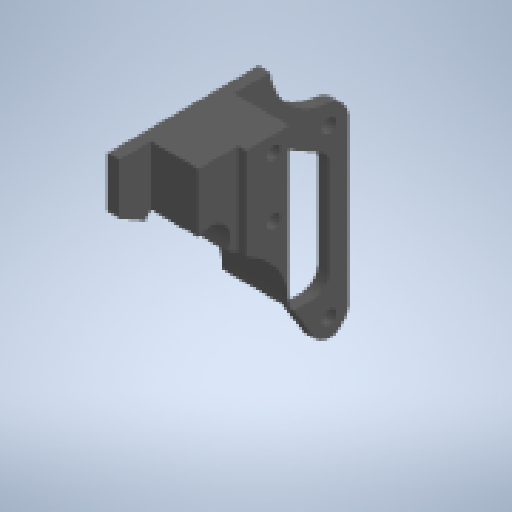
# Autodesk Inventor part: toe_springjoint_bace_upper_left
Saved by Autodesk Inventor 2024.1 (Build 281209000, 209)
## iProperties
Created: 2024-02-25
Part Number: toe_springjoint_bace_upper_left
Material: 一般
Document SubType Name: Modeling
Designer: hibik
Density: 1 g/cm^3
Appearance: 既定
Author: hibik
Autodesk Inventor part; units mm, degrees
ref_plane "YZ Plane" through (0, 0, 0) normal (1, 0, 0) x (0, 1, 0)
ref_plane "XZ Plane" through (0, 0, 0) normal (0, 1, 0) x (-1, 0, 0)
ref_plane "XY Plane" through (0, 0, 0) normal (0, 0, 1) x (1, 0, 0)
sketch "スケッチ1" plane through (0, 0, 0) normal (1, 0, 0) x (0, 1, 0)
  circle A0 centre (0, 0) radius 4.25 construction
  circle A1 centre (0, 0) radius 9
  line L0 (0, 13.5) -> (20, 13.5) construction
  line L1 (20, 13.5) -> (20, -13.5)
  line L2 (20, -13.5) -> (0, -13.5)
  line L3 (0, -13.5) -> (0, 13.5)
  line L4 (20, 5.5) -> (0, 5.5)
  circle A2 centre (0, 0) radius 2.5
  line L5 (0, -2.5) -> (20, -2.5)
  line L6 (20, -2.5) -> (20, -3.5)
  line L7 (20, -3.5) -> (0, -3.5)
  line L8 (0, -3.5) -> (0, -2.5)
  circle A3 centre (39.6712, 2.5) radius 0.8 projected
  line L9 (53.4697, -6.3536) -> (58.9697, 3.1727) projected
  arc A4 (61.7018, 3.9047) -> (58.9697, 3.1727) centre (60.7018, 2.1727) ccw projected
  line L10 (61.7018, 3.9047) -> (71.1182, -1.5319) projected
  arc A5 (71.2169, -4.9351) -> (71.1182, -1.5319) centre (70.1182, -3.2639) ccw projected
  arc A6 (71.2169, -4.9351) -> (66.6149, -12.9061) centre (76.8476, -13.5) ccw projected
  arc A7 (63.6182, -14.5222) -> (66.6149, -12.9061) centre (64.6182, -12.7902) ccw projected
  line L11 (63.6182, -14.5222) -> (54.2018, -9.0857) projected
  arc A8 (53.4697, -6.3536) -> (54.2018, -9.0857) centre (55.2018, -7.3536) ccw projected
  circle A9 centre (63.9111, 6.0933) radius 0.85 projected
  circle A10 centre (71.5976, -22.5933) radius 0.85 projected
  circle A11 centre (10.5, -21) radius 0.85 projected
  circle A12 centre (10.5, 0) radius 0.85 projected
  line L12 (51.6531, -1.5) -> (47.6117, -8.5) projected
  arc A13 (45.8796, -9.5) -> (47.6117, -8.5) centre (45.8796, -7.5) ccw projected
  line L13 (45.8796, -9.5) -> (30.0571, -9.5) projected
  arc A14 (29.2119, -5.6874) -> (30.0571, -9.5) centre (30.0571, -7.5) ccw projected
  line L14 (29.2119, -5.6874) -> (44.2234, 1.3126) projected
  arc A15 (45.0687, 1.5) -> (44.2234, 1.3126) centre (45.0687, -0.5) ccw projected
  line L15 (45.0687, 1.5) -> (49.9211, 1.5) projected
  arc A16 (51.6531, -1.5) -> (49.9211, 1.5) centre (49.9211, -0.5) ccw projected
  circle A17 centre (28.0981, -4) radius 0.8 projected
  circle A18 centre (56.1117, 2.2224) radius 0.8 projected
  line L16 (10.0792, -3.7299) -> (11.4985, -3.068) projected
  arc A19 (14.3437, -4.8806) -> (11.4985, -3.068) centre (12.3437, -4.8806) ccw projected
  line L17 (14.3437, -4.8806) -> (14.3437, -10.4969) projected
  arc A20 (13.5804, -12.0687) -> (14.3437, -10.4969) centre (12.3437, -10.4969) ccw projected
  arc A21 (13.5804, -12.0687) -> (10.5, -15.6905) centre (21, -21.5) ccw projected
  line L18 (10.5, -15.6905) -> (8.0741, -19.9839) projected
  arc A22 (6.3329, -21) -> (8.0741, -19.9839) centre (6.3329, -19) ccw projected
  line L19 (6.3329, -21) -> (-5.5, -21) projected
  arc A23 (-7.5, -19) -> (-5.5, -21) centre (-5.5, -19) ccw projected
  line L20 (-7.5, -19) -> (-7.5, -10.9459) projected
  arc A24 (-4.602, -9.1588) -> (-7.5, -10.9459) centre (-5.5, -10.9459) ccw projected
  arc A25 (-4.602, -9.1588) -> (9.1409, -4.6376) centre (0, 0) ccw projected
  arc A26 (10.0792, -3.7299) -> (9.1409, -4.6376) centre (10.9244, -5.5425) ccw projected
  circle A27 centre (53.4111, -12.0933) radius 0.85 projected
  circle A28 centre (82.0976, -4.4067) radius 0.85 projected
  circle A29 centre (-10.5, -21) radius 0.85 projected
  circle A30 centre (-10.5, 0) radius 0.85 projected
  line L21 (21.7381, 1.5) -> (26.1391, 1.5) projected
  arc A31 (26.9843, -2.3126) -> (26.1391, 1.5) centre (26.1391, -0.5) ccw projected
  line L22 (26.9843, -2.3126) -> (21.189, -5.015) projected
  arc A32 (18.3437, -3.2024) -> (21.189, -5.015) centre (20.3437, -3.2024) ccw projected
  line L23 (18.3437, -3.2024) -> (18.3437, -1.1502) projected
  arc A33 (19.4985, 0.6624) -> (18.3437, -1.1502) centre (20.3437, -1.1502) ccw projected
  line L24 (19.4985, 0.6624) -> (20.8928, 1.3126) projected
  arc A34 (21.7381, 1.5) -> (20.8928, 1.3126) centre (21.7381, -0.5) ccw projected
  circle A35 centre (16.3437, -11.5) radius 0.8 projected
  circle A36 centre (48.189, -11.5) radius 0.8 projected
  arc A37 (10.0455, -23.5) -> (13.0331, -20.7727) centre (10.0455, -20.5) ccw projected
  arc A38 (21, -13.5) -> (13.0331, -20.7727) centre (21, -21.5) ccw projected
  line L25 (21, -13.5) -> (47.704, -13.5) projected
  arc A39 (51.704, -14.5718) -> (47.704, -13.5) centre (47.704, -21.5) ccw projected
  line L26 (51.704, -14.5718) -> (70.0976, -25.1913) projected
  arc A40 (70.0976, -25.1913) -> (83.5976, -1.8087) centre (76.8476, -13.5) ccw projected
  line L27 (83.5976, -1.8087) -> (64.4987, 9.2181) projected
  arc A41 (64.4987, 9.2181) -> (54.7905, 7.895) centre (60.4987, 2.2899) ccw projected
  arc A42 (49.0823, 5.5) -> (54.7905, 7.895) centre (49.0823, 13.5) ccw projected
  line L28 (49.0823, 5.5) -> (16.0857, 5.5) projected
  arc A43 (9.9578, 8.3571) -> (16.0857, 5.5) centre (16.0857, 13.5) ccw projected
  arc A44 (9.9578, 8.3571) -> (-13, 0) centre (0, 0) ccw projected
  line L29 (-13, 0) -> (-13, -20.5) projected
  arc A45 (-13, -20.5) -> (-10, -23.5) centre (-10, -20.5) ccw projected
  line L30 (-10, -23.5) -> (10.0455, -23.5) projected
  circle A46 centre (0, 0) radius 6.25 projected
  circle A47 centre (76.8476, -13.5) radius 6.25 projected
  line L31 (13.5677, 5.5) -> (5.3416, -8.7482)
  circle A48 centre (-10.5, -21) radius 2.2929
  line L32 (-11.6859, -19.0376) -> (5.3416, -8.7482)
  circle A49 centre (10.5, 0) radius 2.5
  line L33 (20, -13.5) -> (20, -13.5627)
  point P0 (8.2916, -3.5)
  point P1 (0, -9)
  point P2 (7.1239, 5.5)
  point P3 (10.5, -2.5)
  point P4 (8.9489, -2.5)
  point P5 (0, -11.976)
  point P6 (12.0557, -13.5)
  point P7 (-7.5, -16.5081)
  point P8 (-12.1213, -22.6213)
  point P9 (11.6684, 2.2102)
  point P10 (20, 0.8963)
  point P11 (20, -5.1726)
  point P12 (8.8095, -1.8418)
  point P13 (8.3716, -3.5)
  point P14 (9.1701, -2.1169)
  point P15 (7.7942, -4.5)
  dimension "d4" = 5
  dimension "d0" = 8.5
  dimension "d2" = 27
  dimension "d3" = 19
  dimension "d5" = 1
  dimension "d8" = 18
  dimension "d11" = 20
  dimension "d12" = 30
  dimension "d13" = 5
  constraints: 24 end point, 7 coincident, 5 point on line, 4 horizontal, 4 parallel, 3 centre point, 2 perpendicular, 2 point on circle, 1 midpoint, 1 tangent, 1 vertical alignment, 7 other
  measures "d0" diameter of A0
  measures "d2" distance of L0.end L1.end
  measures "d3" distance between parallel lines of L2 L4
  measures "d5" distance between parallel lines of L7 L5
  measures "d8" diameter of A1
  measures "d11" distance of L1.end L2.end
  measures "d12" angle of L1 L31
  measures "d13" diameter of A49
extrude "押し出し1" add sketch "スケッチ1" along normal blind 7.5 contours L31 L4 L1 L24 A33 L23 L5 A49 | A49 L5 L31 | L5 L23 A32 L7 A19 L16 L31 | A25 A26 L16 L7 A19 L17 A20 A21 L2 L3 L32 | A1 L31 A25 L3 | L31 L7 L16 A26 A25 | L23 A33 L24 L1 L5 | L5 L1 L7 A32 L23 | A25 L32 L3 | L16 A19 L7 | L7 A32 L1 L2 A21 A20 L17 A19 | L1 A32 L7 | L20 A23 L19 A22 L18 A21 L2 L33 A38 A37 L30 A45 A48 L32 | A48 | A35
sketch "スケッチ3" plane through (7.5, 0, 0) normal (1, 0, 0) x (0, 0, -1)
  line L0 (3.5, 20) -> (3.5, 0) projected
  line L1 (13.5627, 20) -> (-5.5, 20) projected
  line L2 (-5.5, 20) -> (-5.5, 13.5677) projected
  line L3 (9, 0) -> (13.5, 0) projected
  line L4 (13.5, 0) -> (13.5, 12.0557) projected
  line L5 (2.1169, 9.1701) -> (4.5, 7.7942) projected
  line L6 (16.5081, -7.5) -> (19.0376, -11.6859) projected
  arc A0 (13.5, 12.0557) -> (15.6905, 10.5) centre (21.5, 21) ccw projected
  line L7 (15.6905, 10.5) -> (19.9839, 8.0741) projected
  arc A1 (21, 6.3329) -> (19.9839, 8.0741) centre (19, 6.3329) ccw projected
  line L8 (21, 6.3329) -> (21, -5.5) projected
  arc A2 (19, -7.5) -> (21, -5.5) centre (19, -5.5) ccw projected
  line L9 (19, -7.5) -> (16.5081, -7.5) projected
  arc A3 (19.0376, -11.6859) -> (22.6213, -12.1213) centre (21, -10.5) ccw projected
  arc A4 (22.6213, -12.1213) -> (23.5, -10) centre (20.5, -10) ccw projected
  line L10 (23.5, -10) -> (23.5, 10.0455) projected
  arc A5 (23.5, 10.0455) -> (20.7727, 13.0331) centre (20.5, 10.0455) ccw projected
  arc A6 (13.5627, 20) -> (20.7727, 13.0331) centre (21.5, 21) ccw projected
  line L11 (-5.5, 13.5677) -> (-2.2102, 11.6684) projected
  arc A7 (2.1169, 9.1701) -> (-2.2102, 11.6684) centre (0, 10.5) ccw projected
  arc A8 (9, 0) -> (4.5, 7.7942) centre (0, 0) ccw projected
  point P0 (3.5, 20)
  point P1 (3.5, 8.3716)
extrude "押し出し2" add sketch "スケッチ3" along normal blind 1 contours L1 A6 A5 L10 A4 A3 L6 L9 A2 L8 A1 L7 A0 L4 L3 A8 L5 L0
sketch "スケッチ4" plane through (8.5, 0, 0) normal (1, 0, 0) x (0, 0, -1)
  line L0 (9, 0) -> (13.5, 0) projected
  line L1 (13.5, 0) -> (13.5, 12.0557) projected
  arc A0 (13.5, 12.0557) -> (15.6905, 10.5) centre (21.5, 21) ccw projected
  line L2 (15.6905, 10.5) -> (19.9839, 8.0741) projected
  arc A1 (21, 6.3329) -> (19.9839, 8.0741) centre (19, 6.3329) ccw projected
  line L3 (21, 6.3329) -> (21, -5.5) projected
  arc A2 (19, -7.5) -> (21, -5.5) centre (19, -5.5) ccw projected
  line L4 (19, -7.5) -> (16.5081, -7.5) projected
  line L5 (16.5081, -7.5) -> (19.0376, -11.6859) projected
  arc A3 (19.0376, -11.6859) -> (22.6213, -12.1213) centre (21, -10.5) ccw projected
  arc A4 (22.6213, -12.1213) -> (23.5, -10) centre (20.5, -10) ccw projected
  line L6 (23.5, -10) -> (23.5, 10.0455) projected
  arc A5 (23.5, 10.0455) -> (20.7727, 13.0331) centre (20.5, 10.0455) ccw projected
  arc A6 (13.5627, 20) -> (20.7727, 13.0331) centre (21.5, 21) ccw projected
  line L7 (13.5627, 20) -> (3.5, 20) projected
  line L8 (3.5, 20) -> (3.5, 8.3716) projected
  line L9 (3.5, 8.3716) -> (4.5, 7.7942) projected
  arc A7 (9, 0) -> (4.5, 7.7942) centre (0, 0) ccw projected
  line L10 (3.5, 8.3716) -> (3.5, 20) projected
  line L11 (3.5, 20) -> (-5.5, 20) projected
  line L12 (-5.5, 20) -> (-5.5, 13.5677) projected
  line L13 (-5.5, 13.5677) -> (-2.2102, 11.6684) projected
  arc A8 (2.1169, 9.1701) -> (-2.2102, 11.6684) centre (0, 10.5) ccw projected
  line L14 (2.1169, 9.1701) -> (3.5, 8.3716) projected
  line L15 (-1.5, 20) -> (9, 20)
  line L16 (9, 20) -> (9, 0)
  line L17 (9, 0) -> (-1.5, 0)
  line L18 (-1.5, 0) -> (-1.5, 20)
  arc A9 (9, 0) -> (4.5, 7.7942) centre (0, 0) ccw projected
  line L19 (9, 0) -> (13.5, 0) projected
  point P0 (9, 20)
  point P1 (-1.5, 12.5)
  dimension "d14" = 5
  constraints: 8 end point, 2 parallel, 1 collinear, 1 horizontal, 1 perpendicular, 1 point on line, 1 tangent
  measures "d14" distance between parallel lines of L18 L10
extrude "押し出し3" cut sketch "スケッチ4" against normal blind 7 contours L16 L7 A6 A5 L6 A4 A3 L5 L4 A2 L3 A1 L2 A0 L1 L0 | A8 L13 L12 L11 L18
sketch "スケッチ5" plane through (8.5, 0, 0) normal (1, 0, 0) x (0, 0, -1)
  circle A0 centre (7, 18) radius 0.8 projected
  circle A1 centre (7, 10.5) radius 0.8 projected
  point P0 (0, 0)
extrude "押し出し4" cut sketch "スケッチ5" against normal through all
